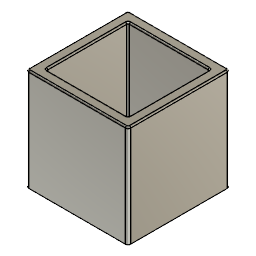
Drip Container (Autodesk Fusion 360 design; units mm, degrees)
Autodesk Fusion 360 part; units mm, degrees
sketch "Sketch1" plane through (0, 0, 0) normal (0, 0, 1) x (1, 0, 0)
  line L0 (75, 75) -> (-75, 75)
  line L1 (-75, 75) -> (-75, -75)
  line L2 (-75, -75) -> (75, -75)
  line L3 (75, -75) -> (75, 75)
  line L4 (75, 75) -> (-75, -75) construction
  line L5 (-75, 75) -> (75, -75) construction
  line L6 (60, 60) -> (-60, 60)
  line L7 (-60, 60) -> (-60, -60)
  line L8 (-60, -60) -> (60, -60)
  line L9 (60, -60) -> (60, 60)
  line L10 (60, 60) -> (-60, -60) construction
  line L11 (-60, 60) -> (60, -60) construction
  dimension "d1" = 150
  dimension "d2" = 150
  dimension "d3" = 120
  dimension "d4" = 120
  constraint horizontal L0
  constraint perpendicular L0 L1
  constraint parallel L0 L2
  constraint parallel L1 L3
  constraint coincident L4 origin
  constraint coincident L5 origin
  constraint horizontal L6
  constraint perpendicular L6 L7
  constraint parallel L6 L8
  constraint parallel L7 L9
  constraint coincident L10 origin
  constraint coincident L11 origin
  measures "d1" distance of L1.end L2.end
  measures "d2" distance of L0.end L1.end
  measures "d3" distance of L7.end L8.end
  measures "d4" distance of L6.end L7.end
extrude "Extrude1" add sketch "Sketch1" along normal blind 10 contours L6 L7 L8 L9
extrude "Extrude2" add sketch "Sketch1" along normal blind 150
fillet "Fillet1" radius 2 12 edges at (-60, 0, 150) (0, 60, 150) (60, 0, 150) (0, -60, 150) (0, 60, 10) (-60, 0, 10) (-60, 60, 80) (0, -60, 10) (-60, -60, 80) (60, -60, 80) (60, 0, 10) (60, 60, 80)
fillet "Fillet2" radius 4 4 edges at (75, -75, 75) (-75, -75, 75) (75, 75, 75) (-75, 75, 75)
fillet "Fillet3" radius 2 8 edges at (-73.8284, 73.8284, 150) (-75, 0, 150) (-73.8284, -73.8284, 150) (0, -75, 150) (73.8284, -73.8284, 150) (75, 0, 150) (73.8284, 73.8284, 150) (0, 75, 150)
